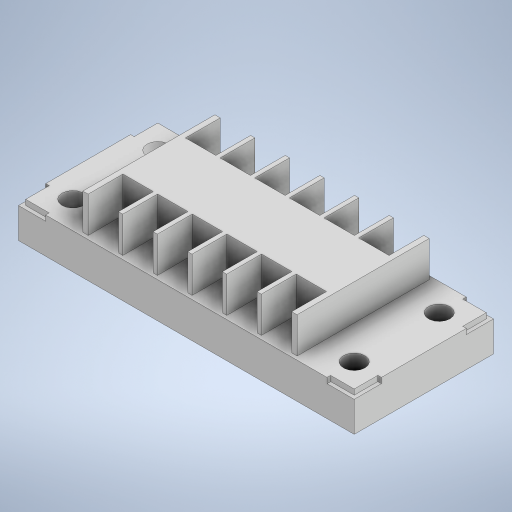
# Autodesk Inventor part: CO-1-01-12VoltFuse
Saved by Autodesk Inventor 2024 (Build 280153000, 153)
## iProperties
Created: 2024-01-25
Part Number: CO-1-01-12VoltFuse
Material: Generic
Document SubType Name: Modeling
Designer: ejned
Density: 1 g/cm^3
Appearance: Default
Author: ejned
Autodesk Inventor part; units mm, degrees
ref_plane "YZ Plane" through (0, 0, 0) normal (1, 0, 0) x (0, 1, 0)
ref_plane "XZ Plane" through (0, 0, 0) normal (0, 1, 0) x (-1, 0, 0)
ref_plane "XY Plane" through (0, 0, 0) normal (0, 0, 1) x (1, 0, 0)
sketch "Sketch1" plane through (0, 0, 0) normal (0, 1, 0) x (-1, 0, 0)
  line L0 (59.69, -24.765) -> (-59.69, -24.765)
  line L1 (-59.69, -24.765) -> (-59.69, 24.765)
  line L2 (-59.69, 24.765) -> (59.69, 24.765)
  line L3 (59.69, 24.765) -> (59.69, -24.765)
  line L4 (59.69, -24.765) -> (-59.69, 24.765) construction
  line L5 (-59.69, -24.765) -> (59.69, 24.765) construction
  point P0 (0, 0)
  dimension "d0" = 119.38
  dimension "d1" = 59.69
  dimension "d2" = 49.53
  dimension "d3" = 24.765
  constraints: 12 end point, 2 midpoint, 2 parallel, 1 horizontal, 1 perpendicular
  measures "d0" distance of L0.start L0.end
  measures "d1" distance from line of point (0, 0) L3
  measures "d2" distance of L2.end L0.start
  measures "d3" distance from line of point (0, 0) L2
extrude "Extrusion1" add sketch "Sketch1" along normal blind 12.7
sketch "Sketch2" plane through (0, 12.7, 0) normal (0, 1, 0) x (1, 0, 0)
  line L0 (38.1, -23.495) -> (-38.1, -23.495)
  line L1 (-38.1, -23.495) -> (-38.1, 23.495)
  line L2 (-38.1, 23.495) -> (38.1, 23.495)
  line L3 (38.1, 23.495) -> (38.1, -23.495)
  line L4 (59.69, -24.765) -> (59.69, 24.765) projected
  line L5 (-59.69, -24.765) -> (59.69, -24.765) projected
  line L6 (-59.69, 24.765) -> (-59.69, -24.765) projected
  point P0 (0, 0)
  dimension "d6" = 21.59
  dimension "d7" = 76.2
  dimension "d8" = 1.27
  dimension "d9" = 46.99
  dimension "d10" = 21.59
  constraints: 8 end point, 2 parallel, 1 horizontal, 1 perpendicular
  measures "d6" distance between parallel lines of L4 L3
  measures "d7" distance of L0.start L0.end
  measures "d8" distance between parallel lines of L0 L5
  measures "d9" distance of L2.end L0.start
  measures "d10" distance between parallel lines of L6 L1
extrude "Extrusion2" add sketch "Sketch2" along normal blind 12.7
sketch "Sketch3" plane through (0, 25.4, 0) normal (0, 1, 0) x (1, 0, 0)
  line L0 (-38.1, 23.495) -> (38.1, 23.495) projected
  line L1 (36.195, 23.495) -> (25.4, 23.495)
  line L2 (25.4, 23.495) -> (25.4, 11.1125)
  line L3 (25.4, 11.1125) -> (36.195, 11.1125)
  line L4 (36.195, 11.1125) -> (36.195, 23.495)
  line L5 (38.1, -23.495) -> (38.1, 23.495) projected
  point P0 (0, 0)
  dimension "d13" = 1.905
  dimension "d14" = 10.795
  dimension "d15" = 11.1125
  constraints: 8 end point, 2 parallel, 1 horizontal, 1 perpendicular, 1 point on line
  measures "d13" distance between parallel lines of L5 L4
  measures "d14" distance between parallel lines of L4 L2
  measures "d15" distance from line of point (0, 0) L3
extrude "Extrusion3" cut sketch "Sketch3" against normal up to surface (12.7 mm away)
pattern_linear "Rectangular Pattern1" count 6 spacing 12.319 along (-1, 0, 0) count 2 spacing -34.6075 along (0, 0, -1) of "Extrusion3"
sketch "Sketch4" plane through (0, 12.7, 0) normal (0, 1, 0) x (1, 0, 0)
  line L0 (-59.69, 24.765) -> (-59.69, -24.765) projected
  line L1 (-59.69, -15.113) -> (-58.42, -15.113)
  line L2 (-58.42, -15.113) -> (-58.42, -23.495)
  line L3 (-58.42, -23.495) -> (-50.038, -23.495)
  line L4 (-50.038, -23.495) -> (-50.038, -24.765)
  line L5 (-50.038, -24.765) -> (-59.69, -24.765)
  line L6 (-59.69, -24.765) -> (-59.69, -15.113)
  line L7 (-59.69, 24.765) -> (-59.69, 15.113)
  line L8 (-59.69, 15.113) -> (-58.42, 15.113)
  line L9 (-58.42, 15.113) -> (-58.42, 23.495)
  line L10 (-58.42, 23.495) -> (-50.038, 23.495)
  line L11 (-50.038, 23.495) -> (-50.038, 24.765)
  line L12 (-50.038, 24.765) -> (-59.69, 24.765)
  point P0 (0, 0)
  dimension "d24" = 1.27
  dimension "d25" = 1.27
  dimension "d26" = 8.382
  dimension "d27" = 1.27
  dimension "d28" = 1.27
  constraints: 24 end point, 9 perpendicular, 6 equal length, 2 point on line, 1 collinear, 1 horizontal
  measures "d24" distance of L3.end L4.end
  measures "d25" distance of L1.start L1.end
  measures "d26" distance between parallel lines of L3 L1
  measures "d27" distance of L7.end L8.end
  measures "d28" distance of L10.end L11.end
extrude "Extrusion4" cut sketch "Sketch4" against normal blind 1.905
mirror "Mirror1" about plane through (0, 0, 0) normal (1, 0, 0) of "Extrusion4"
sketch "Sketch5" plane through (0, 12.7, 0) normal (0, 1, 0) x (1, 0, 0)
  line L0 (-50.038, -24.765) -> (50.038, -24.765) projected
  line L1 (59.69, -15.113) -> (59.69, 15.113) projected
  line L2 (50.038, 24.765) -> (-50.038, 24.765) projected
  point P0 (0, 0)
  point P1 (50.038, -15.113)
  point P2 (50.038, 15.113)
  dimension "d38" = 9.652
  dimension "d39" = 9.652
  dimension "d40" = 9.652
  dimension "d41" = 9.652
  measures "d38" distance from line of point (50.038, -15.113) L0
  measures "d39" distance from line of L1 point (50.038, -15.113)
  measures "d40" distance from line of point (50.038, 15.113) L1
  measures "d41" distance from line of point (50.038, 15.113) L2
hole "Hole1" at (50.038, 12.7, 15.113) at (50.038, 12.7, -15.113) direction (0, -1, 0) diameter 7.62 end through all
mirror "Mirror2" about plane through (0, 0, 0) normal (1, 0, 0) of "Hole1"
body "Solid1"
